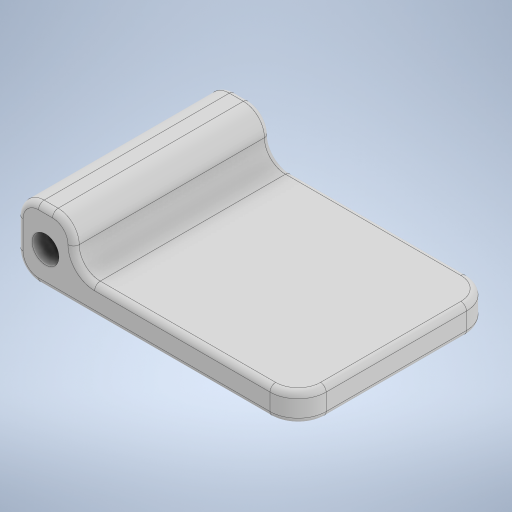
# Autodesk Inventor part: foot rest EG26
Saved by Autodesk Inventor 2023 (Build 270158000, 158)
## iProperties
Created: 2023-10-18
Part Number: foot rest EG26
Material: Generic
Document SubType Name: Modeling
Designer: user
Density: 1 g/cm^3
Appearance: Default
Author: user
Autodesk Inventor part; units mm, degrees
ref_plane "YZ Plane" through (0, 0, 0) normal (1, 0, 0) x (0, 1, 0)
ref_plane "XZ Plane" through (0, 0, 0) normal (0, 1, 0) x (-1, 0, 0)
ref_plane "XY Plane" through (0, 0, 0) normal (0, 0, 1) x (1, 0, 0)
sketch "Sketch1" plane through (0, 0, 0) normal (0, 0, 1) x (1, 0, 0)
  line L0 (0, 0) -> (0, 50)
  line L1 (0, 50) -> (40, 50)
  line L2 (40, 50) -> (40, 20)
  line L3 (40, 20) -> (200, 20)
  line L4 (200, 20) -> (200, 0)
  line L5 (200, 0) -> (0, 0)
  line L6 (20, 50) -> (20, -1.8826)
  line L7 (20, -1.8826) -> (20, 0)
  circle A0 centre (20, 24.0587) radius 9.525
  dimension "d0" = 200
  dimension "d1" = 50
  dimension "d2" = 40
  dimension "d3" = 20
  dimension "d4" = 19.05
  constraints: 16 end point, 6 perpendicular, 2 midpoint, 2 point on line, 1 centre point, 1 vertical
  measures "d0" distance of L4.end L0.start
  measures "d1" distance of L0.start L0.end
  measures "d2" distance of L0.end L1.end
  measures "d3" distance of L3.end L4.end
  measures "d4" diameter of A0
extrude "Extrusion1" add sketch "Sketch1" along normal blind 140 contours L0 L1 L6 A0 L5 | L6 A0 L1 L2 L3 L4 L5
fillet "Fillet1" radius 15 4 edges at (0, 50, 70) (40, 50, 70) (40, 20, 70) (0, 0, 70)
fillet "Fillet2" radius 20 2 edges at (200, 10, 140) (200, 10, 0)
fillet "Fillet3" radius 4 22 edges at (4.3933, 45.6067, 0) (0, 25, 0) (4.3933, 4.3933, 0) (97.4998, 0, 0) (194.1421, 0, 5.8579) (200, 0, 70) (194.1421, 0, 134.1421) (97.4998, 0, 140) (4.3933, 4.3933, 140) (0, 25, 140) (4.3933, 45.6067, 140) (20, 50, 140) (35.6067, 45.6067, 140) (40, 35, 140) (117.4998, 20, 140) (194.1421, 20, 134.1421) (200, 20, 70) (194.1421, 20, 5.8579) (117.4998, 20, 0) (40, 35, 0) (35.6067, 45.6067, 0) (20, 50, 0)
body "Solid1"
